Autodesk Fusion 360 part; units mm, degrees
(part 8 of 18)
  spline S42 degree 5 poles (11.0872, 28.4113) (11.0873, 28.4115) (11.0874, 28.4118) (11.0876, 28.4124) (11.0879, 28.4132) (11.0884, 28.4145) (11.089, 28.4161) (11.0896, 28.4178) (11.0903, 28.4197) (11.0911, 28.4219) (11.0919, 28.4242) (11.0928, 28.4267) (11.0937, 28.4294) (11.0948, 28.4323) (11.0958, 28.4354) (11.0969, 28.4387) (11.0981, 28.4421) (11.0993, 28.4457) (11.1005, 28.4495) (11.1018, 28.4534) (11.1032, 28.4575) (11.1046, 28.4618) (11.106, 28.4662) (11.1074, 28.4708) (11.1089, 28.4755) (11.1105, 28.4804) (11.112, 28.4854) (11.1136, 28.4906) (11.1153, 28.496) (11.1169, 28.5014) (11.1186, 28.5071) (11.1203, 28.5128) (11.1221, 28.5187) (11.1238, 28.5248) (11.1256, 28.531) (11.1274, 28.5373) (11.1293, 28.5437) (11.1311, 28.5503) (11.133, 28.557) (11.1349, 28.5639) (11.1368, 28.5708) (11.1387, 28.5779) (11.1407, 28.5851) (11.1427, 28.5925) (11.1446, 28.6) (11.1466, 28.6075) (11.1486, 28.6153) (11.1507, 28.6231) (11.1527, 28.631) (11.1547, 28.6391) (11.1568, 28.6473) (11.1588, 28.6555) (11.1609, 28.6639) (11.163, 28.6725) (11.1651, 28.6811) (11.1672, 28.6898) (11.1693, 28.6987) (11.1714, 28.7076) (11.1735, 28.7167) (11.1756, 28.7259) (11.1777, 28.7351) (11.1798, 28.7445) (11.1819, 28.754) (11.1841, 28.7636) (11.1862, 28.7733) (11.1883, 28.783) (11.1904, 28.7929) (11.1926, 28.8029) (11.1947, 28.813) (11.1968, 28.8232) (11.1989, 28.8335) (11.201, 28.8438) (11.2032, 28.8543) (11.2053, 28.8649) (11.2074, 28.8755) (11.2095, 28.8863) (11.2116, 28.8971) (11.2137, 28.9081) (11.2158, 28.9191) (11.2179, 28.9302) (11.2199, 28.9415) (11.222, 28.9528) (11.2241, 28.9642) (11.2261, 28.9756) (11.2282, 28.9872) (11.2302, 28.9989) (11.2323, 29.0106) (11.2343, 29.0224) (11.2363, 29.0344) (11.2383, 29.0464) (11.2403, 29.0584) (11.2423, 29.0706) (11.2443, 29.0829) (11.2463, 29.0952) (11.2482, 29.1076) (11.2502, 29.1201) (11.2521, 29.1327) (11.254, 29.1453) (11.2559, 29.1581) (11.2578, 29.1709) (11.2597, 29.1838) (11.2616, 29.1968) (11.2634, 29.2098) (11.2653, 29.223) (11.2671, 29.2362) (11.2689, 29.2495) (11.2707, 29.2628) (11.2725, 29.2763) (11.2742, 29.2898) (11.276, 29.3034) (11.2777, 29.317) (11.2794, 29.3308) (11.2811, 29.3446) (11.2828, 29.3585) (11.2845, 29.3724) (11.2861, 29.3865) (11.2878, 29.4006) (11.2894, 29.4147) (11.291, 29.429) (11.2926, 29.4433) (11.2941, 29.4577) (11.2957, 29.4721) (11.2972, 29.4867) (11.2987, 29.5013) (11.3002, 29.5159) (11.3016, 29.5306) (11.3031, 29.5454) (11.3045, 29.5603) (11.3059, 29.5753) (11.3073, 29.5903) (11.3087, 29.6053) (11.31, 29.6205) (11.3113, 29.6357) (11.3126, 29.6509) (11.3139, 29.6663) (11.3152, 29.6817) (11.3164, 29.6971) (11.3176, 29.7126) (11.3188, 29.7282) (11.32, 29.7439) (11.3211, 29.7596) (11.3222, 29.7754) (11.3234, 29.7912) (11.3244, 29.8071) (11.3255, 29.8231) (11.3265, 29.8391) (11.3275, 29.8552) (11.3285, 29.8714) (11.3295, 29.8876) (11.3304, 29.9038) (11.3313, 29.9202) (11.3322, 29.9366) (11.3331, 29.953) (11.3339, 29.9695) (11.3347, 29.9861) (11.3355, 30.0027) (11.3363, 30.0194) (11.337, 30.0362) (11.3377, 30.053) (11.3384, 30.0698) (11.339, 30.0867) (11.3397, 30.1037) (11.3403, 30.1207) (11.3409, 30.1378) (11.3414, 30.155) (11.3419, 30.1722) (11.3424, 30.1894) (11.3429, 30.2067) (11.3434, 30.2241) (11.3438, 30.2415) (11.3442, 30.259) (11.3445, 30.2765) (11.3449, 30.2941) (11.3452, 30.3117) (11.3455, 30.3294) (11.3457, 30.3472) (11.3459, 30.365) (11.3461, 30.3828) (11.3463, 30.4007) (11.3464, 30.4187) (11.3466, 30.4367) (11.3466, 30.4547) (11.3467, 30.4728) (11.3467, 30.491) (11.3467, 30.5092) (11.3467, 30.5275) (11.3466, 30.5458) (11.3465, 30.5642) (11.3464, 30.5826) (11.3462, 30.601) (11.3461, 30.6195) (11.3458, 30.6381) (11.3456, 30.6567) (11.3453, 30.6754) (11.345, 30.6941) (11.3447, 30.7128) (11.3443, 30.7316) (11.3439, 30.7505) (11.3435, 30.7694) (11.343, 30.7884) (11.3426, 30.8073) (11.342, 30.8264) (11.3415, 30.8455) (11.3409, 30.8646) (11.3403, 30.8838) (11.3397, 30.903) (11.339, 30.9223) (11.3383, 30.9416) (11.3375, 30.961) (11.3368, 30.9804) (11.336, 30.9999) (11.3351, 31.0194) (11.3343, 31.0389) (11.3334, 31.0585) (11.3324, 31.0782) (11.3315, 31.0979) (11.3305, 31.1176) (11.3294, 31.1374) (11.3284, 31.1572) (11.3273, 31.177) (11.3262, 31.1969) (11.325, 31.2169) (11.3238, 31.2369) (11.3226, 31.2569) (11.3213, 31.277) (11.32, 31.2971) (11.3187, 31.3173) (11.3173, 31.3375) (11.3159, 31.3577) (11.3145, 31.378) (11.3131, 31.3983) (11.3116, 31.4187) (11.31, 31.4391) (11.3085, 31.4595) (11.3069, 31.48) (11.3052, 31.5006) (11.3036, 31.5211) (11.3019, 31.5417) (11.3001, 31.5624) (11.2984, 31.5831) (11.2966, 31.6038) (11.2951, 31.6204) (11.294, 31.6329) (11.2932, 31.6412) (11.2929, 31.6454) knots 0 0 0 0 0 0 0.00416667 0.00833333 0.0125 0.01666667 0.02083333 0.025 0.02916667 0.03333333 0.0375 0.04166667 0.04583333 0.05 0.05416667 0.05833333 0.0625 0.06666667 0.07083333 0.075 0.07916667 0.08333333 0.0875 0.09166667 0.09583333 0.1 0.10416667 0.10833333 0.1125 0.11666667 0.12083333 0.125 0.12916667 0.13333333 0.1375 0.14166667 0.14583333 0.15 0.15416667 0.15833333 0.1625 0.16666667 0.17083333 0.175 0.17916667 0.18333333 0.1875 0.19166667 0.19583333 0.2 0.20416667 0.20833333 0.2125 0.21666667 0.22083333 0.225 0.22916667 0.23333333 0.2375 0.24166667 0.24583333 0.25 0.25416667 0.25833333 0.2625 0.26666667 0.27083333 0.275 0.27916667 0.28333333 0.2875 0.29166667 0.29583333 0.3 0.30416667 0.30833333 0.3125 0.31666667 0.32083333 0.325 0.32916667 0.33333333 0.3375 0.34166667 0.34583333 0.35 0.35416667 0.35833333 0.3625 0.36666667 0.37083333 0.375 0.37916667 0.38333333 0.3875 0.39166667 0.39583333 0.4 0.40416667 0.40833333 0.4125 0.41666667 0.42083333 0.425 0.42916667 0.43333333 0.4375 0.44166667 0.44583333 0.45 0.45416667 0.45833333 0.4625 0.46666667 0.47083333 0.475 0.47916667 0.48333333 0.4875 0.49166667 0.49583333 0.5 0.50416667 0.50833333 0.5125 0.51666667 0.52083333 0.525 0.52916667 0.53333333 0.5375 0.54166667 0.54583333 0.55 0.55416667 0.55833333 0.5625 0.56666667 0.57083333 0.575 0.57916667 0.58333333 0.5875 0.59166667 0.59583333 0.6 0.60416667 0.60833333 0.6125 0.61666667 0.62083333 0.625 0.62916667 0.63333333 0.6375 0.64166667 0.64583333 0.65 0.65416667 0.65833333 0.6625 0.66666667 0.67083333 0.675 0.67916667 0.68333333 0.6875 0.69166667 0.69583333 0.7 0.70416667 0.70833333 0.7125 0.71666667 0.72083333 0.725 0.72916667 0.73333333 0.7375 0.74166667 0.74583333 0.75 0.75416667 0.75833333 0.7625 0.76666667 0.77083333 0.775 0.77916667 0.78333333 0.7875 0.79166667 0.79583333 0.8 0.80416667 0.80833333 0.8125 0.81666667 0.82083333 0.825 0.82916667 0.83333333 0.8375 0.84166667 0.84583333 0.85 0.85416667 0.85833333 0.8625 0.86666667 0.87083333 0.875 0.87916667 0.88333333 0.8875 0.89166667 0.89583333 0.9 0.90416667 0.90833333 0.9125 0.91666667 0.92083333 0.925 0.92916667 0.93333333 0.9375 0.94166667 0.94583333 0.95 0.95416667 0.95833333 0.9625 0.96666667 0.97083333 0.975 0.97916667 0.98333333 0.9875 0.99166667 0.99583333 1 1 1 1 1 1
  arc A43 (11.2929, 31.6454) -> (9.4646, 32.2394) centre (0, 0) ccw
  spline S43 degree 5 poles (9.4646, 32.2394) (9.4618, 32.2363) (9.4563, 32.23) (9.4481, 32.2206) (9.4371, 32.208) (9.4235, 32.1923) (9.4099, 32.1766) (9.3964, 32.1609) (9.3829, 32.1452) (9.3694, 32.1295) (9.356, 32.1139) (9.3427, 32.0982) (9.3294, 32.0826) (9.3162, 32.067) (9.303, 32.0514) (9.2899, 32.0358) (9.2768, 32.0203) (9.2638, 32.0047) (9.2508, 31.9892) (9.2379, 31.9736) (9.225, 31.9581) (9.2122, 31.9426) (9.1994, 31.9271) (9.1867, 31.9117) (9.174, 31.8962) (9.1614, 31.8808) (9.1489, 31.8653) (9.1364, 31.8499) (9.1239, 31.8345) (9.1115, 31.8192) (9.0992, 31.8038) (9.0869, 31.7885) (9.0746, 31.7731) (9.0624, 31.7578) (9.0503, 31.7425) (9.0382, 31.7273) (9.0262, 31.712) (9.0142, 31.6968) (9.0023, 31.6816) (8.9904, 31.6664) (8.9786, 31.6512) (8.9668, 31.636) (8.9551, 31.6209) (8.9434, 31.6058) (8.9318, 31.5907) (8.9202, 31.5756) (8.9087, 31.5605) (8.8973, 31.5455) (8.8859, 31.5304) (8.8745, 31.5154) (8.8632, 31.5005) (8.852, 31.4855) (8.8408, 31.4706) (8.8296, 31.4557) (8.8186, 31.4408) (8.8075, 31.4259) (8.7966, 31.4111) (8.7856, 31.3962) (8.7748, 31.3814) (8.7639, 31.3667) (8.7532, 31.3519) (8.7425, 31.3372) (8.7318, 31.3225) (8.7212, 31.3078) (8.7107, 31.2931) (8.7002, 31.2785) (8.6897, 31.2639) (8.6794, 31.2493) (8.669, 31.2348) (8.6587, 31.2202) (8.6485, 31.2057) (8.6383, 31.1912) (8.6282, 31.1768) (8.6182, 31.1624) (8.6082, 31.148) (8.5982, 31.1336) (8.5883, 31.1193) (8.5785, 31.105) (8.5687, 31.0907) (8.5589, 31.0764) (8.5492, 31.0622) (8.5396, 31.048) (8.53, 31.0338) (8.5205, 31.0197) (8.5111, 31.0056) (8.5016, 30.9915) (8.4923, 30.9775) (8.483, 30.9635) (8.4737, 30.9495) (8.4646, 30.9356) (8.4554, 30.9216) (8.4463, 30.9078) (8.4373, 30.8939) (8.4283, 30.8801) (8.4194, 30.8663) (8.4106, 30.8526) (8.4017, 30.8388) (8.393, 30.8252) (8.3843, 30.8115) (8.3757, 30.7979) (8.3671, 30.7843) (8.3585, 30.7708) (8.3501, 30.7573) (8.3416, 30.7438) (8.3333, 30.7304) (8.325, 30.717) (8.3167, 30.7037) (8.3085, 30.6904) (8.3004, 30.6771) (8.2923, 30.6639) (8.2842, 30.6507) (8.2763, 30.6375) (8.2683, 30.6244) (8.2605, 30.6113) (8.2527, 30.5983) (8.2449, 30.5853) (8.2372, 30.5723) (8.2296, 30.5594) (8.222, 30.5466) (8.2145, 30.5337) (8.207, 30.521) (8.1996, 30.5082) (8.1922, 30.4955) (8.1849, 30.4829) (8.1776, 30.4703) (8.1705, 30.4577) (8.1633, 30.4452) (8.1562, 30.4327) (8.1492, 30.4203) (8.1422, 30.408) (8.1353, 30.3956) (8.1285, 30.3834) (8.1217, 30.3711) (8.1149, 30.359) (8.1083, 30.3468) (8.1016, 30.3348) (8.0951, 30.3228) (8.0885, 30.3108) (8.0821, 30.2989) (8.0757, 30.287) (8.0693, 30.2752) (8.063, 30.2634) (8.0568, 30.2517) (8.0506, 30.2401) (8.0445, 30.2285) (8.0385, 30.2169) (8.0325, 30.2054) (8.0265, 30.194) (8.0206, 30.1826) (8.0148, 30.1713) (8.009, 30.1601) (8.0033, 30.1489) (7.9976, 30.1378) (7.992, 30.1267) (7.9865, 30.1157) (7.981, 30.1047) (7.9756, 30.0938) (7.9702, 30.083) (7.9649, 30.0722) (7.9596, 30.0615) (7.9544, 30.0509) (7.9493, 30.0403) (7.9442, 30.0298) (7.9392, 30.0194) (7.9342, 30.0091) (7.9293, 29.9988) (7.9245, 29.9885) (7.9197, 29.9784) (7.9149, 29.9683) (7.9103, 29.9583) (7.9057, 29.9483) (7.9011, 29.9385) (7.8966, 29.9287) (7.8922, 29.919) (7.8878, 29.9093) (7.8834, 29.8998) (7.8792, 29.8903) (7.875, 29.8809) (7.8708, 29.8715) (7.8667, 29.8623) (7.8627, 29.8531) (7.8587, 29.844) (7.8548, 29.835) (7.8509, 29.8261) (7.8471, 29.8173) (7.8434, 29.8085) (7.8397, 29.7999) (7.8361, 29.7913) (7.8325, 29.7828) (7.829, 29.7744) (7.8256, 29.7661) (7.8222, 29.7579) (7.8189, 29.7498) (7.8156, 29.7418) (7.8124, 29.7339) (7.8093, 29.7261) (7.8062, 29.7184) (7.8032, 29.7107) (7.8002, 29.7032) (7.7973, 29.6958) (7.7944, 29.6885) (7.7916, 29.6813) (7.7889, 29.6742) (7.7862, 29.6672) (7.7836, 29.6603) (7.7811, 29.6536) (7.7786, 29.6469) (7.7762, 29.6404) (7.7738, 29.634) (7.7715, 29.6277) (7.7693, 29.6215) (7.7671, 29.6155) (7.765, 29.6095) (7.7629, 29.6037) (7.7609, 29.598) (7.7589, 29.5925) (7.7571, 29.5871) (7.7552, 29.5818) (7.7535, 29.5767) (7.7518, 29.5717) (7.7502, 29.5668) (7.7486, 29.5621) (7.7471, 29.5576) (7.7456, 29.5531) (7.7442, 29.5489) (7.7429, 29.5448) (7.7416, 29.5408) (7.7404, 29.537) (7.7393, 29.5334) (7.7382, 29.53) (7.7372, 29.5267) (7.7363, 29.5236) (7.7354, 29.5206) (7.7345, 29.5179) (7.7338, 29.5153) (7.7331, 29.513) (7.7325, 29.5108) (7.7319, 29.5088) (7.7314, 29.507) (7.7309, 29.5055) (7.7306, 29.5041) (7.7303, 29.5032) (7.7301, 29.5026) (7.7301, 29.5023) (7.73, 29.5021) knots -1 -1 -1 -1 -1 -1 -0.99583333 -0.99166667 -0.9875 -0.98333333 -0.97916667 -0.975 -0.97083333 -0.96666667 -0.9625 -0.95833333 -0.95416667 -0.95 -0.94583333 -0.94166667 -0.9375 -0.93333333 -0.92916667 -0.925 -0.92083333 -0.91666667 -0.9125 -0.90833333 -0.90416667 -0.9 -0.89583333 -0.89166667 -0.8875 -0.88333333 -0.87916667 -0.875 -0.87083333 -0.86666667 -0.8625 -0.85833333 -0.85416667 -0.85 -0.84583333 -0.84166667 -0.8375 -0.83333333 -0.82916667 -0.825 -0.82083333 -0.81666667 -0.8125 -0.80833333 -0.80416667 -0.8 -0.79583333 -0.79166667 -0.7875 -0.78333333 -0.77916667 -0.775 -0.77083333 -0.76666667 -0.7625 -0.75833333 -0.75416667 -0.75 -0.74583333 -0.74166667 -0.7375 -0.73333333 -0.72916667 -0.725 -0.72083333 -0.71666667 -0.7125 -0.70833333 -0.70416667 -0.7 -0.69583333 -0.69166667 -0.6875 -0.68333333 -0.67916667 -0.675 -0.67083333 -0.66666667 -0.6625 -0.65833333 -0.65416667 -0.65 -0.64583333 -0.64166667 -0.6375 -0.63333333 -0.62916667 -0.625 -0.62083333 -0.61666667 -0.6125 -0.60833333 -0.60416667 -0.6 -0.59583333 -0.59166667 -0.5875 -0.58333333 -0.57916667 -0.575 -0.57083333 -0.56666667 -0.5625 -0.55833333 -0.55416667 -0.55 -0.54583333 -0.54166667 -0.5375 -0.53333333 -0.52916667 -0.525 -0.52083333 -0.51666667 -0.5125 -0.50833333 -0.50416667 -0.5 -0.49583333 -0.49166667 -0.4875 -0.48333333 -0.47916667 -0.475 -0.47083333 -0.46666667 -0.4625 -0.45833333 -0.45416667 -0.45 -0.44583333 -0.44166667 -0.4375 -0.43333333 -0.42916667 -0.425 -0.42083333 -0.41666667 -0.4125 -0.40833333 -0.40416667 -0.4 -0.39583333 -0.39166667 -0.3875 -0.38333333 -0.37916667 -0.375 -0.37083333 -0.36666667 -0.3625 -0.35833333 -0.35416667 -0.35 -0.34583333 -0.34166667 -0.3375 -0.33333333 -0.32916667 -0.325 -0.32083333 -0.31666667 -0.3125 -0.30833333 -0.30416667 -0.3 -0.29583333 -0.29166667 -0.2875 -0.28333333 -0.27916667 -0.275 -0.27083333 -0.26666667 -0.2625 -0.25833333 -0.25416667 -0.25 -0.24583333 -0.24166667 -0.2375 -0.23333333 -0.22916667 -0.225 -0.22083333 -0.21666667 -0.2125 -0.20833333 -0.20416667 -0.2 -0.19583333 -0.19166667 -0.1875 -0.18333333 -0.17916667 -0.175 -0.17083333 -0.16666667 -0.1625 -0.15833333 -0.15416667 -0.15 -0.14583333 -0.14166667 -0.1375 -0.13333333 -0.12916667 -0.125 -0.12083333 -0.11666667 -0.1125 -0.10833333 -0.10416667 -0.1 -0.09583333 -0.09166667 -0.0875 -0.08333333 -0.07916667 -0.075 -0.07083333 -0.06666667 -0.0625 -0.05833333 -0.05416667 -0.05 -0.04583333 -0.04166667 -0.0375 -0.03333333 -0.02916667 -0.025 -0.02083333 -0.01666667 -0.0125 -0.00833333 -0.00416667 0 0 0 0 0 0
  line L86 (7.73, 29.5021) -> (7.7297, 29.5008)
  line L87 (7.7297, 29.5008) -> (7.3186, 27.9321)
  arc A44 (7.3186, 27.9321) -> (4.6751, 28.494) centre (0, 0) ccw
  line L88 (4.6751, 28.494) -> (4.9377, 30.0943)
  line L89 (4.9377, 30.0943) -> (4.9379, 30.0956)
  spline S44 degree 5 poles (4.9379, 30.0956) (4.9379, 30.0958) (4.938, 30.0961) (4.9381, 30.0967) (4.9382, 30.0976) (4.9384, 30.099) (4.9386, 30.1006) (4.9389, 30.1025) (4.9392, 30.1045) (4.9395, 30.1068) (4.9398, 30.1092) (4.9401, 30.1119) (4.9405, 30.1147) (4.9409, 30.1177) (4.9413, 30.121) (4.9417, 30.1244) (4.9421, 30.128) (4.9426, 30.1317) (4.943, 30.1357) (4.9434, 30.1398) (4.9439, 30.1441) (4.9444, 30.1486) (4.9448, 30.1532) (4.9453, 30.158) (4.9458, 30.1629) (4.9463, 30.168) (4.9468, 30.1733) (4.9472, 30.1787) (4.9477, 30.1842) (4.9482, 30.1899) (4.9487, 30.1958) (4.9492, 30.2018) (4.9496, 30.2079) (4.9501, 30.2142) (4.9506, 30.2206) (4.951, 30.2272) (4.9515, 30.2339) (4.9519, 30.2407) (4.9524, 30.2477) (4.9528, 30.2547) (4.9532, 30.262) (4.9537, 30.2693) (4.9541, 30.2768) (4.9545, 30.2844) (4.9548, 30.2921) (4.9552, 30.2999) (4.9556, 30.3079) (4.9559, 30.3159) (4.9562, 30.3241) (4.9566, 30.3324) (4.9569, 30.3409) (4.9572, 30.3494) (4.9574, 30.3581) (4.9577, 30.3668) (4.9579, 30.3757) (4.9582, 30.3847) (4.9584, 30.3938) (4.9586, 30.4029) (4.9588, 30.4122) (4.9589, 30.4217) (4.9591, 30.4312) (4.9592, 30.4408) (4.9593, 30.4505) (4.9594, 30.4603) (4.9594, 30.4702) (4.9595, 30.4802) (4.9595, 30.4904) (4.9595, 30.5006) (4.9595, 30.5109) (4.9594, 30.5213) (4.9594, 30.5318) (4.9593, 30.5424) (4.9592, 30.553) (4.9591, 30.5638) (4.9589, 30.5747) (4.9587, 30.5856) (4.9585, 30.5967) (4.9583, 30.6078) (4.9581, 30.6191) (4.9578, 30.6304) (4.9575, 30.6418) (4.9572, 30.6533) (4.9568, 30.6648) (4.9565, 30.6765) (4.9561, 30.6882) (4.9556, 30.7001) (4.9552, 30.712) (4.9547, 30.724) (4.9542, 30.736) (4.9537, 30.7482) (4.9531, 30.7604) (4.9525, 30.7727) (4.9519, 30.7851) (4.9513, 30.7976) (4.9506, 30.8102) (4.9499, 30.8228) (4.9492, 30.8355) (4.9484, 30.8483) (4.9476, 30.8611) (4.9468, 30.8741) (4.946, 30.8871) (4.9451, 30.9002) (4.9442, 30.9133) (4.9433, 30.9265) (4.9423, 30.9398) (4.9413, 30.9532) (4.9403, 30.9667) (4.9393, 30.9802) (4.9382, 30.9938) (4.9371, 31.0074) (4.9359, 31.0211) (4.9347, 31.0349) (4.9335, 31.0488) (4.9323, 31.0627) (4.931, 31.0767) (4.9297, 31.0908) (4.9284, 31.1049) (4.927, 31.1191) (4.9256, 31.1334) (4.9242, 31.1477) (4.9227, 31.1621) (4.9212, 31.1766) (4.9197, 31.1911) (4.9181, 31.2057) (4.9165, 31.2204) (4.9149, 31.2351) (4.9132, 31.2499) (4.9115, 31.2647) (4.9098, 31.2796) (4.908, 31.2946) (4.9063, 31.3096) (4.9044, 31.3247) (4.9026, 31.3398) (4.9006, 31.355) (4.8987, 31.3703) (4.8967, 31.3856) (4.8947, 31.401) (4.8927, 31.4164) (4.8906, 31.4319) (4.8885, 31.4475) (4.8864, 31.4631) (4.8842, 31.4787) (4.882, 31.4945) (4.8797, 31.5103) (4.8774, 31.5261) (4.8751, 31.542) (4.8727, 31.5579) (4.8703, 31.5739) (4.8679, 31.59) (4.8654, 31.6061) (4.8629, 31.6223) (4.8604, 31.6385) (4.8578, 31.6548) (4.8552, 31.6711) (4.8526, 31.6874) (4.8499, 31.7039) (4.8471, 31.7204) (4.8444, 31.7369) (4.8416, 31.7535) (4.8387, 31.7701) (4.8359, 31.7868) (4.833, 31.8035) (4.83, 31.8203) (4.827, 31.8371) (4.824, 31.854) (4.821, 31.871) (4.8179, 31.8879) (4.8147, 31.905) (4.8115, 31.922) (4.8083, 31.9392) (4.8051, 31.9563) (4.8018, 31.9736) (4.7985, 31.9908) (4.7951, 32.0081) (4.7917, 32.0255) (4.7883, 32.0429) (4.7848, 32.0604) (4.7813, 32.0779) (4.7777, 32.0954) (4.7741, 32.113) (4.7705, 32.1306) (4.7668, 32.1483) (4.7631, 32.166) (4.7593, 32.1838) (4.7555, 32.2016) (4.7517, 32.2195) (4.7478, 32.2374) (4.7439, 32.2553) (4.74, 32.2733) (4.736, 32.2913) (4.732, 32.3094) (4.7279, 32.3275) (4.7238, 32.3457) (4.7196, 32.3639) (4.7154, 32.3821) (4.7112, 32.4004) (4.707, 32.4187) (4.7026, 32.4371) (4.6983, 32.4555) (4.6939, 32.4739) (4.6895, 32.4924) (4.685, 32.5109) (4.6805, 32.5295) (4.676, 32.5481) (4.6714, 32.5667) (4.6667, 32.5854) (4.6621, 32.6041) (4.6574, 32.6228) (4.6526, 32.6416) (4.6478, 32.6605) (4.643, 32.6793) (4.6381, 32.6982) (4.6332, 32.7172) (4.6283, 32.7362) (4.6233, 32.7552) (4.6182, 32.7742) (4.6132, 32.7933) (4.608, 32.8125) (4.6029, 32.8316) (4.5977, 32.8508) (4.5924, 32.87) (4.5872, 32.8893) (4.5818, 32.9086) (4.5765, 32.928) (4.5711, 32.9473) (4.5656, 32.9667) (4.5601, 32.9862) (4.5546, 33.0057) (4.549, 33.0252) (4.5434, 33.0447) (4.5378, 33.0643) (4.5321, 33.0839) (4.5263, 33.1036) (4.5206, 33.1232) (4.5147, 33.1429) (4.5089, 33.1627) (4.503, 33.1825) (4.497, 33.2023) (4.491, 33.2221) (4.485, 33.242) (4.4789, 33.2619) (4.474, 33.2778) (4.4703, 33.2898) (4.4679, 33.2978) (4.4666, 33.3018) knots 0 0 0 0 0 0 0.00416667 0.00833333 0.0125 0.01666667 0.02083333 0.025 0.02916667 0.03333333 0.0375 0.04166667 0.04583333 0.05 0.05416667 0.05833333 0.0625 0.06666667 0.07083333 0.075 0.07916667 0.08333333 0.0875 0.09166667 0.09583333 0.1 0.10416667 0.10833333 0.1125 0.11666667 0.12083333 0.125 0.12916667 0.13333333 0.1375 0.14166667 0.14583333 0.15 0.15416667 0.15833333 0.1625 0.16666667 0.17083333 0.175 0.17916667 0.18333333 0.1875 0.19166667 0.19583333 0.2 0.20416667 0.20833333 0.2125 0.21666667 0.22083333 0.225 0.22916667 0.23333333 0.2375 0.24166667 0.24583333 0.25 0.25416667 0.25833333 0.2625 0.26666667 0.27083333 0.275 0.27916667 0.28333333 0.2875 0.29166667 0.29583333 0.3 0.30416667 0.30833333 0.3125 0.31666667 0.32083333 0.325 0.32916667 0.33333333 0.3375 0.34166667 0.34583333 0.35 0.35416667 0.35833333 0.3625 0.36666667 0.37083333 0.375 0.37916667 0.38333333 0.3875 0.39166667 0.39583333 0.4 0.40416667 0.40833333 0.4125 0.41666667 0.42083333 0.425 0.42916667 0.43333333 0.4375 0.44166667 0.44583333 0.45 0.45416667 0.45833333 0.4625 0.46666667 0.47083333 0.475 0.47916667 0.48333333 0.4875 0.49166667 0.49583333 0.5 0.50416667 0.50833333 0.5125 0.51666667 0.52083333 0.525 0.52916667 0.53333333 0.5375 0.54166667 0.54583333 0.55 0.55416667 0.55833333 0.5625 0.56666667 0.57083333 0.575 0.57916667 0.58333333 0.5875 0.59166667 0.59583333 0.6 0.60416667 0.60833333 0.6125 0.61666667 0.62083333 0.625 0.62916667 0.63333333 0.6375 0.64166667 0.64583333 0.65 0.65416667 0.65833333 0.6625 0.66666667 0.67083333 0.675 0.67916667 0.68333333 0.6875 0.69166667 0.69583333 0.7 0.70416667 0.70833333 0.7125 0.71666667 0.72083333 0.725 0.72916667 0.73333333 0.7375 0.74166667 0.74583333 0.75 0.75416667 0.75833333 0.7625 0.76666667 0.77083333 0.775 0.77916667 0.78333333 0.7875 0.79166667 0.79583333 0.8 0.80416667 0.80833333 0.8125 0.81666667 0.82083333 0.825 0.82916667 0.83333333 0.8375 0.84166667 0.84583333 0.85 0.85416667 0.85833333 0.8625 0.86666667 0.87083333 0.875 0.87916667 0.88333333 0.8875 0.89166667 0.89583333 0.9 0.90416667 0.90833333 0.9125 0.91666667 0.92083333 0.925 0.92916667 0.93333333 0.9375 0.94166667 0.94583333 0.95 0.95416667 0.95833333 0.9625 0.96666667 0.97083333 0.975 0.97916667 0.98333333 0.9875 0.99166667 0.99583333 1 1 1 1 1 1
  arc A45 (4.4666, 33.3018) -> (2.5548, 33.5027) centre (0, 0) ccw
  spline S45 degree 5 poles (2.5548, 33.5027) (2.5528, 33.4991) (2.5487, 33.4918) (2.5426, 33.4808) (2.5345, 33.4662) (2.5244, 33.448) (2.5144, 33.4299) (2.5044, 33.4117) (2.4945, 33.3936) (2.4846, 33.3754) (2.4747, 33.3574) (2.4649, 33.3393) (2.4552, 33.3212) (2.4455, 33.3032) (2.4359, 33.2852) (2.4262, 33.2672) (2.4167, 33.2493) (2.4072, 33.2314) (2.3977, 33.2135) (2.3883, 33.1956) (2.379, 33.1777) (2.3696, 33.1599) (2.3604, 33.1421) (2.3512, 33.1243) (2.342, 33.1066) (2.3329, 33.0889) (2.3238, 33.0712) (2.3147, 33.0535) (2.3058, 33.0358) (2.2968, 33.0182) (2.2879, 33.0006) (2.2791, 32.9831) (2.2703, 32.9655) (2.2616, 32.948) (2.2529, 32.9306) (2.2442, 32.9131) (2.2356, 32.8957) (2.2271, 32.8783) (2.2186, 32.8609) (2.2101, 32.8436) (2.2017, 32.8263) (2.1933, 32.809) (2.185, 32.7918) (2.1768, 32.7745) (2.1685, 32.7573) (2.1604, 32.7402) (2.1522, 32.7231) (2.1442, 32.706) (2.1361, 32.6889) (2.1282, 32.6719) (2.1202, 32.6549) (2.1123, 32.6379) (2.1045, 32.621) (2.0967, 32.6041) (2.089, 32.5872) (2.0813, 32.5704) (2.0736, 32.5536) (2.066, 32.5368) (2.0584, 32.52) (2.0509, 32.5033) (2.0435, 32.4867) (2.0361, 32.47) (2.0287, 32.4534) (2.0214, 32.4369) (2.0141, 32.4203) (2.0069, 32.4039) (1.9997, 32.3874) (1.9926, 32.371) (1.9855, 32.3546) (1.9785, 32.3382) (1.9715, 32.3219) (1.9646, 32.3057) (1.9577, 32.2894) (1.9508, 32.2732) (1.944, 32.2571) (1.9373, 32.2409) (1.9306, 32.2248) (1.9239, 32.2088) (1.9173, 32.1928) (1.9107, 32.1768) (1.9042, 32.1609) (1.8978, 32.145) (1.8913, 32.1292) (1.885, 32.1134) (1.8786, 32.0976) (1.8724, 32.0819) (1.8661, 32.0662) (1.8599, 32.0506) (1.8538, 32.035) (1.8477, 32.0194) (1.8417, 32.0039) (1.8357, 31.9884) (1.8297, 31.973) (1.8238, 31.9576) (1.818, 31.9423) (1.8122, 31.927) (1.8064, 31.9118) (1.8007, 31.8966) (1.795, 31.8814) (1.7894, 31.8663) (1.7838, 31.8512) (1.7783, 31.8362) (1.7728, 31.8213) (1.7673, 31.8063) (1.762, 31.7915) (1.7566, 31.7766) (1.7513, 31.7619) (1.7461, 31.7471) (1.7409, 31.7325) (1.7357, 31.7178) (1.7306, 31.7033) (1.7255, 31.6887) (1.7205, 31.6743) (1.7155, 31.6598) (1.7106, 31.6455) (1.7057, 31.6311) (1.7009, 31.6169) (1.6961, 31.6027) (1.6913, 31.5885) (1.6866, 31.5744) (1.682, 31.5603) (1.6774, 31.5463) (1.6728, 31.5324) (1.6683, 31.5185) (1.6638, 31.5047) (1.6594, 31.4909) (1.655, 31.4772) (1.6507, 31.4635) (1.6464, 31.4499) (1.6421, 31.4363) (1.6379, 31.4229) (1.6338, 31.4094) (1.6297, 31.3961) (1.6256, 31.3827) (1.6216, 31.3695) (1.6176, 31.3563) (1.6137, 31.3432) (1.6098, 31.3301) (1.606, 31.3171) (1.6022, 31.3042) (1.5984, 31.2913) (1.5947, 31.2785) (1.5911, 31.2657) (1.5875, 31.2531) (1.5839, 31.2405) (1.5804, 31.2279) (1.5769, 31.2154) (1.5734, 31.203) (1.57, 31.1907) (1.5667, 31.1784) (1.5634, 31.1662) (1.5601, 31.154) (1.5569, 31.142) (1.5537, 31.13) (1.5506, 31.1181) (1.5475, 31.1062) (1.5444, 31.0944) (1.5414, 31.0827) (1.5385, 31.0711) (1.5356, 31.0595) (1.5327, 31.0481) (1.5299, 31.0366) (1.5271, 31.0253) (1.5243, 31.0141) (1.5216, 31.0029) (1.519, 30.9918) (1.5163, 30.9808) (1.5138, 30.9699) (1.5112, 30.959) (1.5087, 30.9483) (1.5063, 30.9376) (1.5039, 30.927) (1.5015, 30.9165) (1.4992, 30.906) (1.4969, 30.8957) (1.4947, 30.8854) (1.4925, 30.8753) (1.4903, 30.8652) (1.4882, 30.8552) (1.4861, 30.8453) (1.4841, 30.8355) (1.4821, 30.8258) (1.4801, 30.8162) (1.4782, 30.8066) (1.4763, 30.7972) (1.4745, 30.7879) (1.4727, 30.7787) (1.4709, 30.7695) (1.4692, 30.7605) (1.4675, 30.7516) (1.4659, 30.7427) (1.4643, 30.734) (1.4627, 30.7254) (1.4612, 30.7169) (1.4597, 30.7084) (1.4582, 30.7001) (1.4568, 30.6919) (1.4554, 30.6839) (1.4541, 30.6759) (1.4528, 30.668) (1.4515, 30.6603) (1.4503, 30.6527) (1.4491, 30.6452) (1.4479, 30.6378) (1.4468, 30.6305) (1.4457, 30.6234) (1.4447, 30.6163) (1.4437, 30.6094) (1.4427, 30.6027) (1.4417, 30.596) (1.4408, 30.5895) (1.4399, 30.5832) (1.4391, 30.5769) (1.4383, 30.5708) (1.4375, 30.5648) (1.4368, 30.559) (1.4361, 30.5533) (1.4354, 30.5478) (1.4347, 30.5424) (1.4341, 30.5372) (1.4335, 30.5321) (1.4329, 30.5271) (1.4324, 30.5224) (1.4319, 30.5177) (1.4314, 30.5133) (1.431, 30.509) (1.4306, 30.5049) (1.4302, 30.5009) (1.4298, 30.4971) (1.4295, 30.4935) (1.4292, 30.4901) (1.4289, 30.4869) (1.4286, 30.4838) (1.4284, 30.481) (1.4282, 30.4783) (1.428, 30.4758) (1.4278, 30.4736) (1.4277, 30.4715) (1.4276, 30.4697) (1.4275, 30.468) (1.4274, 30.4667) (1.4273, 30.4657) (1.4273, 30.4651) (1.4273, 30.4648) (1.4273, 30.4646) knots -1 -1 -1 -1 -1 -1 -0.99583333 -0.99166667 -0.9875 -0.98333333 -0.97916667 -0.975 -0.97083333 -0.96666667 -0.9625 -0.95833333 -0.95416667 -0.95 -0.94583333 -0.94166667 -0.9375 -0.93333333 -0.92916667 -0.925 -0.92083333 -0.91666667 -0.9125 -0.90833333 -0.90416667 -0.9 -0.89583333 -0.89166667 -0.8875 -0.88333333 -0.87916667 -0.875 -0.87083333 -0.86666667 -0.8625 -0.85833333 -0.85416667 -0.85 -0.84583333 -0.84166667 -0.8375 -0.83333333 -0.82916667 -0.825 -0.82083333 -0.81666667 -0.8125 -0.80833333 -0.80416667 -0.8 -0.79583333 -0.79166667 -0.7875 -0.78333333 -0.77916667 -0.775 -0.77083333 -0.76666667 -0.7625 -0.75833333 -0.75416667 -0.75 -0.74583333 -0.74166667 -0.7375 -0.73333333 -0.72916667 -0.725 -0.72083333 -0.71666667 -0.7125 -0.70833333 -0.70416667 -0.7 -0.69583333 -0.69166667 -0.6875 -0.68333333 -0.67916667 -0.675 -0.67083333 -0.66666667 -0.6625 -0.65833333 -0.65416667 -0.65 -0.64583333 -0.64166667 -0.6375 -0.63333333 -0.62916667 -0.625 -0.62083333 -0.61666667 -0.6125 -0.60833333 -0.60416667 -0.6 -0.59583333 -0.59166667 -0.5875 -0.58333333 -0.57916667 -0.575 -0.57083333 -0.56666667 -0.5625 -0.55833333 -0.55416667 -0.55 -0.54583333 -0.54166667 -0.5375 -0.53333333 -0.52916667 -0.525 -0.52083333 -0.51666667 -0.5125 -0.50833333 -0.50416667 -0.5 -0.49583333 -0.49166667 -0.4875 -0.48333333 -0.47916667 -0.475 -0.47083333 -0.46666667 -0.4625 -0.45833333 -0.45416667 -0.45 -0.44583333 -0.44166667 -0.4375 -0.43333333 -0.42916667 -0.425 -0.42083333 -0.41666667 -0.4125 -0.40833333 -0.40416667 -0.4 -0.39583333 -0.39166667 -0.3875 -0.38333333 -0.37916667 -0.375 -0.37083333 -0.36666667 -0.3625 -0.35833333 -0.35416667 -0.35 -0.34583333 -0.34166667 -0.3375 -0.33333333 -0.32916667 -0.325 -0.32083333 -0.31666667 -0.3125 -0.30833333 -0.30416667 -0.3 -0.29583333 -0.29166667 -0.2875 -0.28333333 -0.27916667 -0.275 -0.27083333 -0.26666667 -0.2625 -0.25833333 -0.25416667 -0.25 -0.24583333 -0.24166667 -0.2375 -0.23333333 -0.22916667 -0.225 -0.22083333 -0.21666667 -0.2125 -0.20833333 -0.20416667 -0.2 -0.19583333 -0.19166667 -0.1875 -0.18333333 -0.17916667 -0.175 -0.17083333 -0.16666667 -0.1625 -0.15833333 -0.15416667 -0.15 -0.14583333 -0.14166667 -0.1375 -0.13333333 -0.12916667 -0.125 -0.12083333 -0.11666667 -0.1125 -0.10833333 -0.10416667 -0.1 -0.09583333 -0.09166667 -0.0875 -0.08333333 -0.07916667 -0.075 -0.07083333 -0.06666667 -0.0625 -0.05833333 -0.05416667 -0.05 -0.04583333 -0.04166667 -0.0375 -0.03333333 -0.02916667 -0.025 -0.02083333 -0.01666667 -0.0125 -0.00833333 -0.00416667 0 0 0 0 0 0
  line L90 (1.4273, 30.4646) -> (1.4272, 30.4632)
  line L91 (1.4272, 30.4632) -> (1.3513, 28.8434)
  arc A46 (1.3513, 28.8434) -> (-1.3513, 28.8434) centre (0, 0) ccw
  line L92 (-1.3513, 28.8434) -> (-1.4272, 30.4632)
  line L93 (-1.4272, 30.4632) -> (-1.4273, 30.4646)
  spline S46 degree 5 poles (-1.4273, 30.4646) (-1.4273, 30.4648) (-1.4273, 30.4651) (-1.4273, 30.4657) (-1.4274, 30.4667) (-1.4275, 30.468) (-1.4276, 30.4697) (-1.4277, 30.4715) (-1.4278, 30.4736) (-1.428, 30.4758) (-1.4282, 30.4783) (-1.4284, 30.481) (-1.4286, 30.4838) (-1.4289, 30.4869) (-1.4292, 30.4901) (-1.4295, 30.4935) (-1.4298, 30.4971) (-1.4302, 30.5009) (-1.4306, 30.5049) (-1.431, 30.509) (-1.4314, 30.5133) (-1.4319, 30.5177) (-1.4324, 30.5224) (-1.4329, 30.5271) (-1.4335, 30.5321) (-1.4341, 30.5372) (-1.4347, 30.5424) (-1.4354, 30.5478) (-1.4361, 30.5533) (-1.4368, 30.559) (-1.4375, 30.5648) (-1.4383, 30.5708) (-1.4391, 30.5769) (-1.4399, 30.5832) (-1.4408, 30.5895) (-1.4417, 30.596) (-1.4427, 30.6027) (-1.4437, 30.6094) (-1.4447, 30.6163) (-1.4457, 30.6234) (-1.4468, 30.6305) (-1.4479, 30.6378) (-1.4491, 30.6452) (-1.4503, 30.6527) (-1.4515, 30.6603) (-1.4528, 30.668) (-1.4541, 30.6759) (-1.4554, 30.6839) (-1.4568, 30.6919) (-1.4582, 30.7001) (-1.4597, 30.7084) (-1.4612, 30.7169) (-1.4627, 30.7254) (-1.4643, 30.734) (-1.4659, 30.7427) (-1.4675, 30.7516) (-1.4692, 30.7605) (-1.4709, 30.7695) (-1.4727, 30.7787) (-1.4745, 30.7879) (-1.4763, 30.7972) (-1.4782, 30.8066) (-1.4801, 30.8162) (-1.4821, 30.8258) (-1.4841, 30.8355) (-1.4861, 30.8453) (-1.4882, 30.8552) (-1.4903, 30.8652) (-1.4925, 30.8753) (-1.4947, 30.8854) (-1.4969, 30.8957) (-1.4992, 30.906) (-1.5015, 30.9165) (-1.5039, 30.927) (-1.5063, 30.9376) (-1.5087, 30.9483) (-1.5112, 30.959) (-1.5138, 30.9699) (-1.5163, 30.9808) (-1.519, 30.9918) (-1.5216, 31.0029) (-1.5243, 31.0141) (-1.5271, 31.0253) (-1.5299, 31.0366) (-1.5327, 31.0481) (-1.5356, 31.0595) (-1.5385, 31.0711) (-1.5414, 31.0827) (-1.5444, 31.0944) (-1.5475, 31.1062) (-1.5506, 31.1181) (-1.5537, 31.13) (-1.5569, 31.142) (-1.5601, 31.154) (-1.5634, 31.1662) (-1.5667, 31.1784) (-1.57, 31.1907) (-1.5734, 31.203) (-1.5769, 31.2154) (-1.5804, 31.2279) (-1.5839, 31.2405) (-1.5875, 31.2531) (-1.5911, 31.2657) (-1.5947, 31.2785) (-1.5984, 31.2913) (-1.6022, 31.3042) (-1.606, 31.3171) (-1.6098, 31.3301) (-1.6137, 31.3432) (-1.6176, 31.3563) (-1.6216, 31.3695) (-1.6256, 31.3827) (-1.6297, 31.3961) (-1.6338, 31.4094) (-1.6379, 31.4229) (-1.6421, 31.4363) (-1.6464, 31.4499) (-1.6507, 31.4635) (-1.655, 31.4772) (-1.6594, 31.4909) (-1.6638, 31.5047) (-1.6683, 31.5185) (-1.6728, 31.5324) (-1.6774, 31.5463) (-1.682, 31.5603) (-1.6866, 31.5744) (-1.6913, 31.5885) (-1.6961, 31.6027) (-1.7009, 31.6169) (-1.7057, 31.6311) (-1.7106, 31.6455) (-1.7155, 31.6598) (-1.7205, 31.6743) (-1.7255, 31.6887) (-1.7306, 31.7033) (-1.7357, 31.7178) (-1.7409, 31.7325) (-1.7461, 31.7471) (-1.7513, 31.7619) (-1.7566, 31.7766) (-1.762, 31.7915) (-1.7673, 31.8063) (-1.7728, 31.8213) (-1.7783, 31.8362) (-1.7838, 31.8512) (-1.7894, 31.8663) (-1.795, 31.8814) (-1.8007, 31.8966) (-1.8064, 31.9118) (-1.8122, 31.927) (-1.818, 31.9423) (-1.8238, 31.9576) (-1.8297, 31.973) (-1.8357, 31.9884) (-1.8417, 32.0039) (-1.8477, 32.0194) (-1.8538, 32.035) (-1.8599, 32.0506) (-1.8661, 32.0662) (-1.8724, 32.0819) (-1.8786, 32.0976) (-1.885, 32.1134) (-1.8913, 32.1292) (-1.8978, 32.145) (-1.9042, 32.1609) (-1.9107, 32.1768) (-1.9173, 32.1928) (-1.9239, 32.2088) (-1.9306, 32.2248) (-1.9373, 32.2409) (-1.944, 32.2571) (-1.9508, 32.2732) (-1.9577, 32.2894) (-1.9646, 32.3057) (-1.9715, 32.3219) (-1.9785, 32.3382) (-1.9855, 32.3546) (-1.9926, 32.371) (-1.9997, 32.3874) (-2.0069, 32.4039) (-2.0141, 32.4203) (-2.0214, 32.4369) (-2.0287, 32.4534) (-2.0361, 32.47) (-2.0435, 32.4867) (-2.0509, 32.5033) (-2.0584, 32.52) (-2.066, 32.5368) (-2.0736, 32.5536) (-2.0813, 32.5704) (-2.089, 32.5872) (-2.0967, 32.6041) (-2.1045, 32.621) (-2.1123, 32.6379) (-2.1202, 32.6549) (-2.1282, 32.6719) (-2.1361, 32.6889) (-2.1442, 32.706) (-2.1522, 32.7231) (-2.1604, 32.7402) (-2.1685, 32.7573) (-2.1768, 32.7745) (-2.185, 32.7918) (-2.1933, 32.809) (-2.2017, 32.8263) (-2.2101, 32.8436) (-2.2186, 32.8609) (-2.2271, 32.8783) (-2.2356, 32.8957) (-2.2442, 32.9131) (-2.2529, 32.9306) (-2.2616, 32.948) (-2.2703, 32.9655) (-2.2791, 32.9831) (-2.2879, 33.0006) (-2.2968, 33.0182) (-2.3058, 33.0358) (-2.3147, 33.0535) (-2.3238, 33.0712) (-2.3329, 33.0889) (-2.342, 33.1066) (-2.3512, 33.1243) (-2.3604, 33.1421) (-2.3696, 33.1599) (-2.379, 33.1777) (-2.3883, 33.1956) (-2.3977, 33.2135) (-2.4072, 33.2314) (-2.4167, 33.2493) (-2.4262, 33.2672) (-2.4359, 33.2852) (-2.4455, 33.3032) (-2.4552, 33.3212) (-2.4649, 33.3393) (-2.4747, 33.3574) (-2.4846, 33.3754) (-2.4945, 33.3936) (-2.5044, 33.4117) (-2.5144, 33.4299) (-2.5244, 33.448) (-2.5345, 33.4662) (-2.5426, 33.4808) (-2.5487, 33.4918) (-2.5528, 33.4991) (-2.5548, 33.5027) knots 0 0 0 0 0 0 0.00416667 0.00833333 0.0125 0.01666667 0.02083333 0.025 0.02916667 0.03333333 0.0375 0.04166667 0.04583333 0.05 0.05416667 0.05833333 0.0625 0.06666667 0.07083333 0.075 0.07916667 0.08333333 0.0875 0.09166667 0.09583333 0.1 0.10416667 0.10833333 0.1125 0.11666667 0.12083333 0.125 0.12916667 0.13333333 0.1375 0.14166667 0.14583333 0.15 0.15416667 0.15833333 0.1625 0.16666667 0.17083333 0.175 0.17916667 0.18333333 0.1875 0.19166667 0.19583333 0.2 0.20416667 0.20833333 0.2125 0.21666667 0.22083333 0.225 0.22916667 0.23333333 0.2375 0.24166667 0.24583333 0.25 0.25416667 0.25833333 0.2625 0.26666667 0.27083333 0.275 0.27916667 0.28333333 0.2875 0.29166667 0.29583333 0.3 0.30416667 0.30833333 0.3125 0.31666667 0.32083333 0.325 0.32916667 0.33333333 0.3375 0.34166667 0.34583333 0.35 0.35416667 0.35833333 0.3625 0.36666667 0.37083333 0.375 0.37916667 0.38333333 0.3875 0.39166667 0.39583333 0.4 0.40416667 0.40833333 0.4125 0.41666667 0.42083333 0.425 0.42916667 0.43333333 0.4375 0.44166667 0.44583333 0.45 0.45416667 0.45833333 0.4625 0.46666667 0.47083333 0.475 0.47916667 0.48333333 0.4875 0.49166667 0.49583333 0.5 0.50416667 0.50833333 0.5125 0.51666667 0.52083333 0.525 0.52916667 0.53333333 0.5375 0.54166667 0.54583333 0.55 0.55416667 0.55833333 0.5625 0.56666667 0.57083333 0.575 0.57916667 0.58333333 0.5875 0.59166667 0.59583333 0.6 0.60416667 0.60833333 0.6125 0.61666667 0.62083333 0.625 0.62916667 0.63333333 0.6375 0.64166667 0.64583333 0.65 0.65416667 0.65833333 0.6625 0.66666667 0.67083333 0.675 0.67916667 0.68333333 0.6875 0.69166667 0.69583333 0.7 0.70416667 0.70833333 0.7125 0.71666667 0.72083333 0.725 0.72916667 0.73333333 0.7375 0.74166667 0.74583333 0.75 0.75416667 0.75833333 0.7625 0.76666667 0.77083333 0.775 0.77916667 0.78333333 0.7875 0.79166667 0.79583333 0.8 0.80416667 0.80833333 0.8125 0.81666667 0.82083333 0.825 0.82916667 0.83333333 0.8375 0.84166667 0.84583333 0.85 0.85416667 0.85833333 0.8625 0.86666667 0.87083333 0.875 0.87916667 0.88333333 0.8875 0.89166667 0.89583333 0.9 0.90416667 0.90833333 0.9125 0.91666667 0.92083333 0.925 0.92916667 0.93333333 0.9375 0.94166667 0.94583333 0.95 0.95416667 0.95833333 0.9625 0.96666667 0.97083333 0.975 0.97916667 0.98333333 0.9875 0.99166667 0.99583333 1 1 1 1 1 1
  arc A47 (-2.5548, 33.5027) -> (-4.4666, 33.3018) centre (0, 0) ccw
  spline S47 degree 5 poles (-4.4666, 33.3018) (-4.4679, 33.2978) (-4.4703, 33.2898) (-4.474, 33.2778) (-4.4789, 33.2619) (-4.485, 33.242) (-4.491, 33.2221) (-4.497, 33.2023) (-4.503, 33.1825) (-4.5089, 33.1627) (-4.5147, 33.1429) (-4.5206, 33.1232) (-4.5263, 33.1036) (-4.5321, 33.0839) (-4.5378, 33.0643) (-4.5434, 33.0447) (-4.549, 33.0252) (-4.5546, 33.0057) (-4.5601, 32.9862) (-4.5656, 32.9667) (-4.5711, 32.9473) (-4.5765, 32.928) (-4.5818, 32.9086) (-4.5872, 32.8893) (-4.5924, 32.87) (-4.5977, 32.8508) (-4.6029, 32.8316) (-4.608, 32.8125) (-4.6132, 32.7933) (-4.6182, 32.7742) (-4.6233, 32.7552) (-4.6283, 32.7362) (-4.6332, 32.7172) (-4.6381, 32.6982) (-4.643, 32.6793) (-4.6478, 32.6605) (-4.6526, 32.6416) (-4.6574, 32.6228) (-4.6621, 32.6041) (-4.6667, 32.5854) (-4.6714, 32.5667) (-4.676, 32.5481) (-4.6805, 32.5295) (-4.685, 32.5109) (-4.6895, 32.4924) (-4.6939, 32.4739) (-4.6983, 32.4555) (-4.7026, 32.4371) (-4.707, 32.4187) (-4.7112, 32.4004) (-4.7154, 32.3821) (-4.7196, 32.3639) (-4.7238, 32.3457) (-4.7279, 32.3275) (-4.732, 32.3094) (-4.736, 32.2913) (-4.74, 32.2733) (-4.7439, 32.2553) (-4.7478, 32.2374) (-4.7517, 32.2195) (-4.7555, 32.2016) (-4.7593, 32.1838) (-4.7631, 32.166) (-4.7668, 32.1483) (-4.7705, 32.1306) (-4.7741, 32.113) (-4.7777, 32.0954) (-4.7813, 32.0779) (-4.7848, 32.0604) (-4.7883, 32.0429) (-4.7917, 32.0255) (-4.7951, 32.0081) (-4.7985, 31.9908) (-4.8018, 31.9736) (-4.8051, 31.9563) (-4.8083, 31.9392) (-4.8115, 31.922) (-4.8147, 31.905) (-4.8179, 31.8879) (-4.821, 31.871) (-4.824, 31.854) (-4.827, 31.8371) (-4.83, 31.8203) (-4.833, 31.8035) (-4.8359, 31.7868) (-4.8387, 31.7701) (-4.8416, 31.7535) (-4.8444, 31.7369) (-4.8471, 31.7204) (-4.8499, 31.7039) (-4.8526, 31.6874) (-4.8552, 31.6711) (-4.8578, 31.6548) (-4.8604, 31.6385) (-4.8629, 31.6223) (-4.8654, 31.6061) (-4.8679, 31.59) (-4.8703, 31.5739) (-4.8727, 31.5579) (-4.8751, 31.542) (-4.8774, 31.5261) (-4.8797, 31.5103) (-4.882, 31.4945) (-4.8842, 31.4787) (-4.8864, 31.4631) (-4.8885, 31.4475) (-4.8906, 31.4319) (-4.8927, 31.4164) (-4.8947, 31.401) (-4.8967, 31.3856) (-4.8987, 31.3703) (-4.9006, 31.355) (-4.9026, 31.3398) (-4.9044, 31.3247) (-4.9063, 31.3096) (-4.908, 31.2946) (-4.9098, 31.2796) (-4.9115, 31.2647) (-4.9132, 31.2499) (-4.9149, 31.2351) (-4.9165, 31.2204) (-4.9181, 31.2057) (-4.9197, 31.1911) (-4.9212, 31.1766) (-4.9227, 31.1621) (-4.9242, 31.1477) (-4.9256, 31.1334) (-4.927, 31.1191) (-4.9284, 31.1049) (-4.9297, 31.0908) (-4.931, 31.0767) (-4.9323, 31.0627) (-4.9335, 31.0488) (-4.9347, 31.0349) (-4.9359, 31.0211) (-4.9371, 31.0074) (-4.9382, 30.9938) (-4.9393, 30.9802) (-4.9403, 30.9667) (-4.9413, 30.9532) (-4.9423, 30.9398) (-4.9433, 30.9265) (-4.9442, 30.9133) (-4.9451, 30.9002) (-4.946, 30.8871) (-4.9468, 30.8741) (-4.9476, 30.8611) (-4.9484, 30.8483) (-4.9492, 30.8355) (-4.9499, 30.8228) (-4.9506, 30.8102) (-4.9513, 30.7976) (-4.9519, 30.7851) (-4.9525, 30.7727) (-4.9531, 30.7604) (-4.9537, 30.7482) (-4.9542, 30.736) (-4.9547, 30.724) (-4.9552, 30.712) (-4.9556, 30.7001) (-4.9561, 30.6882) (-4.9565, 30.6765) (-4.9568, 30.6648) (-4.9572, 30.6533) (-4.9575, 30.6418) (-4.9578, 30.6304) (-4.9581, 30.6191) (-4.9583, 30.6078) (-4.9585, 30.5967) (-4.9587, 30.5856) (-4.9589, 30.5747) (-4.9591, 30.5638) (-4.9592, 30.553) (-4.9593, 30.5424) (-4.9594, 30.5318) (-4.9594, 30.5213) (-4.9595, 30.5109) (-4.9595, 30.5006) (-4.9595, 30.4904) (-4.9595, 30.4802) (-4.9594, 30.4702) (-4.9594, 30.4603) (-4.9593, 30.4505) (-4.9592, 30.4408) (-4.9591, 30.4312) (-4.9589, 30.4217) (-4.9588, 30.4122) (-4.9586, 30.4029) (-4.9584, 30.3938) (-4.9582, 30.3847) (-4.9579, 30.3757) (-4.9577, 30.3668) (-4.9574, 30.3581) (-4.9572, 30.3494) (-4.9569, 30.3409) (-4.9566, 30.3324) (-4.9562, 30.3241) (-4.9559, 30.3159) (-4.9556, 30.3079) (-4.9552, 30.2999) (-4.9548, 30.2921) (-4.9545, 30.2844) (-4.9541, 30.2768) (-4.9537, 30.2693) (-4.9532, 30.262) (-4.9528, 30.2547) (-4.9524, 30.2477) (-4.9519, 30.2407) (-4.9515, 30.2339) (-4.951, 30.2272) (-4.9506, 30.2206) (-4.9501, 30.2142) (-4.9496, 30.2079) (-4.9492, 30.2018) (-4.9487, 30.1958) (-4.9482, 30.1899) (-4.9477, 30.1842) (-4.9472, 30.1787) (-4.9468, 30.1733) (-4.9463, 30.168) (-4.9458, 30.1629) (-4.9453, 30.158) (-4.9448, 30.1532) (-4.9444, 30.1486) (-4.9439, 30.1441) (-4.9434, 30.1398) (-4.943, 30.1357) (-4.9426, 30.1317) (-4.9421, 30.128) (-4.9417, 30.1244) (-4.9413, 30.121) (-4.9409, 30.1177) (-4.9405, 30.1147) (-4.9401, 30.1119) (-4.9398, 30.1092) (-4.9395, 30.1068) (-4.9392, 30.1045) (-4.9389, 30.1025) (-4.9386, 30.1006) (-4.9384, 30.099) (-4.9382, 30.0976) (-4.9381, 30.0967) (-4.938, 30.0961) (-4.9379, 30.0958) (-4.9379, 30.0956) knots -1 -1 -1 -1 -1 -1 -0.99583333 -0.99166667 -0.9875 -0.98333333 -0.97916667 -0.975 -0.97083333 -0.96666667 -0.9625 -0.95833333 -0.95416667 -0.95 -0.94583333 -0.94166667 -0.9375 -0.93333333 -0.92916667 -0.925 -0.92083333 -0.91666667 -0.9125 -0.90833333 -0.90416667 -0.9 -0.89583333 -0.89166667 -0.8875 -0.88333333 -0.87916667 -0.875 -0.87083333 -0.86666667 -0.8625 -0.85833333 -0.85416667 -0.85 -0.84583333 -0.84166667 -0.8375 -0.83333333 -0.82916667 -0.825 -0.82083333 -0.81666667 -0.8125 -0.80833333 -0.80416667 -0.8 -0.79583333 -0.79166667 -0.7875 -0.78333333 -0.77916667 -0.775 -0.77083333 -0.76666667 -0.7625 -0.75833333 -0.75416667 -0.75 -0.74583333 -0.74166667 -0.7375 -0.73333333 -0.72916667 -0.725 -0.72083333 -0.71666667 -0.7125 -0.70833333 -0.70416667 -0.7 -0.69583333 -0.69166667 -0.6875 -0.68333333 -0.67916667 -0.675 -0.67083333 -0.66666667 -0.6625 -0.65833333 -0.65416667 -0.65 -0.64583333 -0.64166667 -0.6375 -0.63333333 -0.62916667 -0.625 -0.62083333 -0.61666667 -0.6125 -0.60833333 -0.60416667 -0.6 -0.59583333 -0.59166667 -0.5875 -0.58333333 -0.57916667 -0.575 -0.57083333 -0.56666667 -0.5625 -0.55833333 -0.55416667 -0.55 -0.54583333 -0.54166667 -0.5375 -0.53333333 -0.52916667 -0.525 -0.52083333 -0.51666667 -0.5125 -0.50833333 -0.50416667 -0.5 -0.49583333 -0.49166667 -0.4875 -0.48333333 -0.47916667 -0.475 -0.47083333 -0.46666667 -0.4625 -0.45833333 -0.45416667 -0.45 -0.44583333 -0.44166667 -0.4375 -0.43333333 -0.42916667 -0.425 -0.42083333 -0.41666667 -0.4125 -0.40833333 -0.40416667 -0.4 -0.39583333 -0.39166667 -0.3875 -0.38333333 -0.37916667 -0.375 -0.37083333 -0.36666667 -0.3625 -0.35833333 -0.35416667 -0.35 -0.34583333 -0.34166667 -0.3375 -0.33333333 -0.32916667 -0.325 -0.32083333 -0.31666667 -0.3125 -0.30833333 -0.30416667 -0.3 -0.29583333 -0.29166667 -0.2875 -0.28333333 -0.27916667 -0.275 -0.27083333 -0.26666667 -0.2625 -0.25833333 -0.25416667 -0.25 -0.24583333 -0.24166667 -0.2375 -0.23333333 -0.22916667 -0.225 -0.22083333 -0.21666667 -0.2125 -0.20833333 -0.20416667 -0.2 -0.19583333 -0.19166667 -0.1875 -0.18333333 -0.17916667 -0.175 -0.17083333 -0.16666667 -0.1625 -0.15833333 -0.15416667 -0.15 -0.14583333 -0.14166667 -0.1375 -0.13333333 -0.12916667 -0.125 -0.12083333 -0.11666667 -0.1125 -0.10833333 -0.10416667 -0.1 -0.09583333 -0.09166667 -0.0875 -0.08333333 -0.07916667 -0.075 -0.07083333 -0.06666667 -0.0625 -0.05833333 -0.05416667 -0.05 -0.04583333 -0.04166667 -0.0375 -0.03333333 -0.02916667 -0.025 -0.02083333 -0.01666667 -0.0125 -0.00833333 -0.00416667 0 0 0 0 0 0
  line L94 (-4.9379, 30.0956) -> (-4.9377, 30.0943)
  line L95 (-4.9377, 30.0943) -> (-4.6751, 28.494)
  arc A48 (-4.6751, 28.494) -> (-7.3186, 27.9321) centre (0, 0) ccw
  line L96 (-7.3186, 27.9321) -> (-7.7297, 29.5008)
  line L97 (-7.7297, 29.5008) -> (-7.73, 29.5021)
  spline S48 degree 5 poles (-7.73, 29.5021) (-7.7301, 29.5023) (-7.7301, 29.5026) (-7.7303, 29.5032) (-7.7306, 29.5041) (-7.7309, 29.5055) (-7.7314, 29.507) (-7.7319, 29.5088) (-7.7325, 29.5108) (-7.7331, 29.513) (-7.7338, 29.5153) (-7.7345, 29.5179) (-7.7354, 29.5206) (-7.7363, 29.5236) (-7.7372, 29.5267) (-7.7382, 29.53) (-7.7393, 29.5334) (-7.7404, 29.537) (-7.7416, 29.5408) (-7.7429, 29.5448) (-7.7442, 29.5489) (-7.7456, 29.5531) (-7.7471, 29.5576) (-7.7486, 29.5621) (-7.7502, 29.5668) (-7.7518, 29.5717) (-7.7535, 29.5767) (-7.7552, 29.5818) (-7.7571, 29.5871) (-7.7589, 29.5925) (-7.7609, 29.598) (-7.7629, 29.6037) (-7.765, 29.6095) (-7.7671, 29.6155) (-7.7693, 29.6215) (-7.7715, 29.6277) (-7.7738, 29.634) (-7.7762, 29.6404) (-7.7786, 29.6469) (-7.7811, 29.6536) (-7.7836, 29.6603) (-7.7862, 29.6672) (-7.7889, 29.6742) (-7.7916, 29.6813) (-7.7944, 29.6885) (-7.7973, 29.6958) (-7.8002, 29.7032) (-7.8032, 29.7107) (-7.8062, 29.7184) (-7.8093, 29.7261) (-7.8124, 29.7339) (-7.8156, 29.7418) (-7.8189, 29.7498) (-7.8222, 29.7579) (-7.8256, 29.7661) (-7.829, 29.7744) (-7.8325, 29.7828) (-7.8361, 29.7913) (-7.8397, 29.7999) (-7.8434, 29.8085) (-7.8471, 29.8173) (-7.8509, 29.8261) (-7.8548, 29.835) (-7.8587, 29.844) (-7.8627, 29.8531) (-7.8667, 29.8623) (-7.8708, 29.8715) (-7.875, 29.8809) (-7.8792, 29.8903) (-7.8834, 29.8998) (-7.8878, 29.9093) (-7.8922, 29.919) (-7.8966, 29.9287) (-7.9011, 29.9385) (-7.9057, 29.9483) (-7.9103, 29.9583) (-7.9149, 29.9683) (-7.9197, 29.9784) (-7.9245, 29.9885) (-7.9293, 29.9988) (-7.9342, 30.0091) (-7.9392, 30.0194) (-7.9442, 30.0298) (-7.9493, 30.0403) (-7.9544, 30.0509) (-7.9596, 30.0615) (-7.9649, 30.0722) (-7.9702, 30.083) (-7.9756, 30.0938) (-7.981, 30.1047) (-7.9865, 30.1157) (-7.992, 30.1267) (-7.9976, 30.1378) (-8.0033, 30.1489) (-8.009, 30.1601) (-8.0148, 30.1713) (-8.0206, 30.1826) (-8.0265, 30.194) (-8.0325, 30.2054) (-8.0385, 30.2169) (-8.0445, 30.2285) (-8.0506, 30.2401) (-8.0568, 30.2517) (-8.063, 30.2634) (-8.0693, 30.2752) (-8.0757, 30.287) (-8.0821, 30.2989) (-8.0885, 30.3108) (-8.0951, 30.3228) (-8.1016, 30.3348) (-8.1083, 30.3468) (-8.1149, 30.359) (-8.1217, 30.3711) (-8.1285, 30.3834) (-8.1353, 30.3956) (-8.1422, 30.408) (-8.1492, 30.4203) (-8.1562, 30.4327) (-8.1633, 30.4452) (-8.1705, 30.4577) (-8.1776, 30.4703) (-8.1849, 30.4829) (-8.1922, 30.4955) (-8.1996, 30.5082) (-8.207, 30.521) (-8.2145, 30.5337) (-8.222, 30.5466) (-8.2296, 30.5594) (-8.2372, 30.5723) (-8.2449, 30.5853) (-8.2527, 30.5983) (-8.2605, 30.6113) (-8.2683, 30.6244) (-8.2763, 30.6375) (-8.2842, 30.6507) (-8.2923, 30.6639) (-8.3004, 30.6771) (-8.3085, 30.6904) (-8.3167, 30.7037) (-8.325, 30.717) (-8.3333, 30.7304) (-8.3416, 30.7438) (-8.3501, 30.7573) (-8.3585, 30.7708) (-8.3671, 30.7843) (-8.3757, 30.7979) (-8.3843, 30.8115) (-8.393, 30.8252) (-8.4017, 30.8388) (-8.4106, 30.8526) (-8.4194, 30.8663) (-8.4283, 30.8801) (-8.4373, 30.8939) (-8.4463, 30.9078) (-8.4554, 30.9216) (-8.4646, 30.9356) (-8.4737, 30.9495) (-8.483, 30.9635) (-8.4923, 30.9775) (-8.5016, 30.9915) (-8.5111, 31.0056) (-8.5205, 31.0197) (-8.53, 31.0338) (-8.5396, 31.048) (-8.5492, 31.0622) (-8.5589, 31.0764) (-8.5687, 31.0907) (-8.5785, 31.105) (-8.5883, 31.1193) (-8.5982, 31.1336) (-8.6082, 31.148) (-8.6182, 31.1624) (-8.6282, 31.1768) (-8.6383, 31.1912) (-8.6485, 31.2057) (-8.6587, 31.2202) (-8.669, 31.2348) (-8.6794, 31.2493) (-8.6897, 31.2639) (-8.7002, 31.2785) (-8.7107, 31.2931) (-8.7212, 31.3078) (-8.7318, 31.3225) (-8.7425, 31.3372) (-8.7532, 31.3519) (-8.7639, 31.3667) (-8.7748, 31.3814) (-8.7856, 31.3962) (-8.7966, 31.4111) (-8.8075, 31.4259) (-8.8186, 31.4408) (-8.8296, 31.4557) (-8.8408, 31.4706) (-8.852, 31.4855) (-8.8632, 31.5005) (-8.8745, 31.5154) (-8.8859, 31.5304) (-8.8973, 31.5455) (-8.9087, 31.5605) (-8.9202, 31.5756) (-8.9318, 31.5907) (-8.9434, 31.6058) (-8.9551, 31.6209) (-8.9668, 31.636) (-8.9786, 31.6512) (-8.9904, 31.6664) (-9.0023, 31.6816) (-9.0142, 31.6968) (-9.0262, 31.712) (-9.0382, 31.7273) (-9.0503, 31.7425) (-9.0624, 31.7578) (-9.0746, 31.7731) (-9.0869, 31.7885) (-9.0992, 31.8038) (-9.1115, 31.8192) (-9.1239, 31.8345) (-9.1364, 31.8499) (-9.1489, 31.8653) (-9.1614, 31.8808) (-9.174, 31.8962) (-9.1867, 31.9117) (-9.1994, 31.9271) (-9.2122, 31.9426) (-9.225, 31.9581) (-9.2379, 31.9736) (-9.2508, 31.9892) (-9.2638, 32.0047) (-9.2768, 32.0203) (-9.2899, 32.0358) (-9.303, 32.0514) (-9.3162, 32.067) (-9.3294, 32.0826) (-9.3427, 32.0982) (-9.356, 32.1139) (-9.3694, 32.1295) (-9.3829, 32.1452) (-9.3964, 32.1609) (-9.4099, 32.1766) (-9.4235, 32.1923) (-9.4371, 32.208) (-9.4481, 32.2206) (-9.4563, 32.23) (-9.4618, 32.2363) (-9.4646, 32.2394) knots 0 0 0 0 0 0 0.00416667 0.00833333 0.0125 0.01666667 0.02083333 0.025 0.02916667 0.03333333 0.0375 0.04166667 0.04583333 0.05 0.05416667 0.05833333 0.0625 0.06666667 0.07083333 0.075 0.07916667 0.08333333 0.0875 0.09166667 0.09583333 0.1 0.10416667 0.10833333 0.1125 0.11666667 0.12083333 0.125 0.12916667 0.13333333 0.1375 0.14166667 0.14583333 0.15 0.15416667 0.15833333 0.1625 0.16666667 0.17083333 0.175 0.17916667 0.18333333 0.1875 0.19166667 0.19583333 0.2 0.20416667 0.20833333 0.2125 0.21666667 0.22083333 0.225 0.22916667 0.23333333 0.2375 0.24166667 0.24583333 0.25 0.25416667 0.25833333 0.2625 0.26666667 0.27083333 0.275 0.27916667 0.28333333 0.2875 0.29166667 0.29583333 0.3 0.30416667 0.30833333 0.3125 0.31666667 0.32083333 0.325 0.32916667 0.33333333 0.3375 0.34166667 0.34583333 0.35 0.35416667 0.35833333 0.3625 0.36666667 0.37083333 0.375 0.37916667 0.38333333 0.3875 0.39166667 0.39583333 0.4 0.40416667 0.40833333 0.4125 0.41666667 0.42083333 0.425 0.42916667 0.43333333 0.4375 0.44166667 0.44583333 0.45 0.45416667 0.45833333 0.4625 0.46666667 0.47083333 0.475 0.47916667 0.48333333 0.4875 0.49166667 0.49583333 0.5 0.50416667 0.50833333 0.5125 0.51666667 0.52083333 0.525 0.52916667 0.53333333 0.5375 0.54166667 0.54583333 0.55 0.55416667 0.55833333 0.5625 0.56666667 0.57083333 0.575 0.57916667 0.58333333 0.5875 0.59166667 0.59583333 0.6 0.60416667 0.60833333 0.6125 0.61666667 0.62083333 0.625 0.62916667 0.63333333 0.6375 0.64166667 0.64583333 0.65 0.65416667 0.65833333 0.6625 0.66666667 0.67083333 0.675 0.67916667 0.68333333 0.6875 0.69166667 0.69583333 0.7 0.70416667 0.70833333 0.7125 0.71666667 0.72083333 0.725 0.72916667 0.73333333 0.7375 0.74166667 0.74583333 0.75 0.75416667 0.75833333 0.7625 0.76666667 0.77083333 0.775 0.77916667 0.78333333 0.7875 0.79166667 0.79583333 0.8 0.80416667 0.80833333 0.8125 0.81666667 0.82083333 0.825 0.82916667 0.83333333 0.8375 0.84166667 0.84583333 0.85 0.85416667 0.85833333 0.8625 0.86666667 0.87083333 0.875 0.87916667 0.88333333 0.8875 0.89166667 0.89583333 0.9 0.90416667 0.90833333 0.9125 0.91666667 0.92083333 0.925 0.92916667 0.93333333 0.9375 0.94166667 0.94583333 0.95 0.95416667 0.95833333 0.9625 0.96666667 0.97083333 0.975 0.97916667 0.98333333 0.9875 0.99166667 0.99583333 1 1 1 1 1 1
  arc A49 (-9.4646, 32.2394) -> (-11.2929, 31.6454) centre (0, 0) ccw